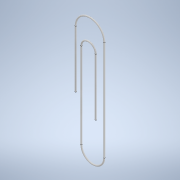
# Autodesk Inventor part: Paper Clip
Saved by Autodesk Inventor 2020 (Build 240168000, 168)
## iProperties
Created: 2020-01-31
Part Number: Paper Clip
Material: Generic
Document SubType Name: Modeling
Designer: cks4a449
Density: 1 g/cm^3
Appearance: Default
Author: cks4a449
Autodesk Inventor part; units mm, degrees
ref_plane "YZ Plane" through (0, 0, 0) normal (1, 0, 0) x (0, 1, 0)
ref_plane "XZ Plane" through (0, 0, 0) normal (0, 1, 0) x (-1, 0, 0)
ref_plane "XY Plane" through (0, 0, 0) normal (0, 0, 1) x (1, 0, 0)
sketch "Sketch1" plane through (0, 0, 0) normal (0, 0, 1) x (1, 0, 0)
  line L0 (0, 0) -> (0, 25.4)
  arc A0 (12.7, 25.4) -> (0, 25.4) centre (6.35, 25.4) ccw
  line L1 (12.7, 25.4) -> (12.7, -19.05)
  arc A1 (2.54, -19.05) -> (12.7, -19.05) centre (7.62, -19.05) ccw
  line L2 (2.54, -19.05) -> (2.54, 19.05)
  arc A2 (8.89, 19.05) -> (2.54, 19.05) centre (5.715, 19.05) ccw
  line L3 (8.89, 19.05) -> (8.89, -6.35)
  dimension "d0" = 25.4
  dimension "d2" = 12.7
  dimension "d3" = 6.35
  dimension "d4" = 44.45
  dimension "d5" = 10.16
  dimension "d7" = 5.08
  dimension "d8" = 38.1
  dimension "d9" = 6.35
  dimension "d10" = 25.4
  constraints: 8 end point, 6 point on circle, 4 vertical, 3 centre point, 1 tangent
  measures "d0" distance of L0.start L0.end
  measures "d2" distance of L0.end L1.start
  measures "d3" radius of A0
  measures "d4" distance of L1.start L1.end
  measures "d5" distance of L1.end L2.start
  measures "d7" radius of A1
  measures "d8" distance of L2.start L2.end
  measures "d9" distance of L2.end L3.start
  measures "d10" distance of L3.start L3.end
sketch "Sketch2" plane through (0, 0, 0) normal (0, 1, 0) x (-1, 0, 0)
  circle A0 centre (0, 0) radius 0.3175
  dimension "d11" = 0.635
  constraints: 1 centre point, 1 coincident
  measures "d11" diameter of A0
sweep "Sweep1" add profiles "Sketch2" path "Sketch1"
body "Solid1"
